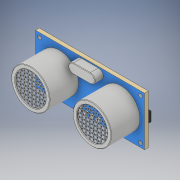
# Autodesk Inventor part: HC-SR04
Saved by Autodesk Inventor 2019 (Build 230136000, 136)
## iProperties
Created: 2020-12-06
Part Number: HC-SR04
Material: Типовые
Document SubType Name: Modeling
Designer: Professional
Density: 1 g/cm^3
Appearance: По умолчанию
Author: Professional
Autodesk Inventor part; units mm, degrees
note: some values were not read from the file. Chosen so that the rebuilt part matches the saved one: sketch regions of "Выдавливание1".
ref_plane "YZ Plane" through (0, 0, 0) normal (1, 0, 0) x (0, 1, 0)
ref_plane "XZ Plane" through (0, 0, 0) normal (0, 1, 0) x (-1, 0, 0)
ref_plane "XY Plane" through (0, 0, 0) normal (0, 0, 1) x (1, 0, 0)
sketch "Эскиз1" plane through (0, 0, 0) normal (0, 0, 1) x (1, 0, 0)
  line L0 (-22.7, -10.2) -> (22.7, -10.2)
  line L1 (22.7, -10.2) -> (22.7, 10.2)
  line L2 (22.7, 10.2) -> (-22.7, 10.2)
  line L3 (-22.7, 10.2) -> (-22.7, -10.2)
  line L4 (0, -10.2) -> (0, 10.2)
  circle A0 centre (-21, 8.5) radius 0.8
  circle A1 centre (-21, -8.5) radius 0.8
  circle A2 centre (21, 8.5) radius 0.8
  circle A3 centre (21, -8.5) radius 0.8
  line L5 (-22.7, 0) -> (22.7, 0)
  point P0 (0, 0)
  dimension "d0" = 45.4
  dimension "d1" = 20.4
  dimension "d2" = 42
  dimension "d3" = 17
  dimension "d4" = 1.6
  constraints: 12 end point, 4 centre point, 4 midpoint, 2 parallel, 2 symmetric about line, 2 vertical alignment, 1 horizontal, 1 horizontal alignment, 1 perpendicular, 1 vertical, 3 other
  measures "d0" distance of L1.end L2.end
  measures "d1" distance between parallel lines of L0 L2
  measures "d2" diameter of A0.centre L4
  measures "d3" distance of A1.centre A0.centre
  measures "d4" diameter of A0
extrude "Выдавливание1" add sketch "Эскиз1" along normal blind 1.6
sketch "Эскиз2" plane through (0, 0, 1.6) normal (0, 0, 1) x (1, 0, 0)
  circle A0 centre (-12.8, 0) radius 8
  circle A1 centre (12.8, 0) radius 8
  line L0 (22.7, 10.2) -> (-22.7, 10.2) projected
  line L1 (0, 10.2) -> (0, -10.2)
  line L2 (-22.7, -10.2) -> (22.7, -10.2) projected
  point P0 (0, 0)
  point P1 (0, 0)
  dimension "d7" = 16
  dimension "d8" = 25.6
  constraints: 3 midpoint, 2 centre point, 2 end point, 1 horizontal alignment, 1 vertical, 1 other
  measures "d7" diameter of A1
  measures "d8" distance of A0.centre A1.centre
extrude "Выдавливание2" add sketch "Эскиз2" along normal blind 12
sketch "Эскиз3" plane through (-12.8, 0, 13.6) normal (0, 0, 1) x (1, 0, 0)
  circle A0 centre (0, 0) radius 6.4
  circle A1 centre (25.6, 0) radius 6.4
  circle A2 centre (25.6, 0) radius 8 projected
  circle A3 centre (0, 0) radius 8 projected
  point P0 (12.8, 0)
  dimension "d11" = 1.6
  constraints: 2 centre point, 2 coincident, 1 equal radius
  measures "d11" radial gap between concentric circles of A2 A1
extrude "Выдавливание3" cut sketch "Эскиз3" against normal blind 0.4 contours A0 | A1
chamfer "Фаска1" distance 0.2 angle 45 4 edges at (-20.8, 0, 13.6) (4.8, 0, 13.6) (-19.2, 0, 13.6) (6.4, 0, 13.6)
sketch "Эскиз4" plane through (0, 0, 1.6) normal (0, 0, 1) x (1, 0, 0)
  line L0 (3.5, 7.7) -> (-3.5, 7.7) construction
  line L1 (3.5, 9.7) -> (-3.5, 9.7)
  line L2 (-3.5, 5.7) -> (3.5, 5.7)
  arc A0 (3.5, 5.7) -> (3.5, 9.7) centre (3.5, 7.7) ccw
  arc A1 (-3.5, 9.7) -> (-3.5, 5.7) centre (-3.5, 7.7) ccw
  line L3 (22.7, 10.2) -> (-22.7, 10.2) projected
  point P0 (0, 0)
  point P1 (0, 7.7)
  dimension "d17" = 7
  dimension "d18" = 2
  dimension "d19" = 2.5
  constraints: 8 end point, 4 point on circle, 4 tangent, 2 centre point, 1 horizontal, 1 midpoint, 1 parallel, 1 vertical alignment
  measures "d17" distance of L0.start L0.end
  measures "d18" radius of A1
  measures "d19" distance between parallel lines of L3 L0
extrude "Выдавливание4" add sketch "Эскиз4" along normal blind 3.5
sketch "Эскиз5" plane through (0, 0, 1.6) normal (0, 0, 1) x (1, 0, 0)
  circle A0 centre (3.81, -8.7) radius 0.8
  circle A1 centre (1.27, -8.7) radius 0.8
  circle A2 centre (-1.27, -8.7) radius 0.8
  circle A3 centre (-3.81, -8.7) radius 0.8
  line L0 (0, 0) -> (0, -10.2)
  line L1 (-22.7, -10.2) -> (22.7, -10.2) projected
  dimension "d22" = 2.54
  dimension "d23" = 7.62
  dimension "d24" = 1.6
  dimension "d25" = 1.5
  constraints: 4 centre point, 2 end point, 1 equal radius, 1 horizontal alignment, 1 midpoint, 2 other
  measures "d22" distance of A2.centre A1.centre
  measures "d23" distance of A3.centre A0.centre
  measures "d24" diameter of A3
  measures "d25" distance from line of L1 A1.centre
extrude "Выдавливание5" add sketch "Эскиз5" along normal blind 1
fillet "Сопряжение1" radius 0.4 4 edges at (-4.61, -8.7, 2.6) (-2.07, -8.7, 2.6) (0.47, -8.7, 2.6) (3.01, -8.7, 2.6)
sketch "Эскиз7" plane through (0, 0, 0) normal (0, 0, -1) x (-1, 0, 0)
  line L0 (-22.2, 2) -> (-13.2, 2)
  line L1 (-13.2, 2) -> (-13.2, -2)
  line L2 (-13.2, -2) -> (-22.2, -2)
  line L3 (-22.2, -2) -> (-22.2, 2)
  line L4 (20.7, 4.5) -> (16.7, 4.5)
  line L5 (16.7, 4.5) -> (16.7, -4.5)
  line L6 (16.7, -4.5) -> (20.7, -4.5)
  line L7 (20.7, -4.5) -> (20.7, 4.5)
  line L8 (-4.5, 2) -> (4.5, 2)
  line L9 (4.5, 2) -> (4.5, -2)
  line L10 (4.5, -2) -> (-4.5, -2)
  line L11 (-4.5, -2) -> (-4.5, 2)
  line L12 (22.7, 10.2) -> (22.7, -10.2) projected
  line L13 (-22.7, -10.2) -> (-22.7, 10.2) projected
  point P0 (0, 0)
  point P1 (0, -2)
  point P2 (-4.5, 0)
  point P3 (16.7, 0)
  dimension "d31" = 9
  dimension "d32" = 4
  dimension "d33" = 2
  dimension "d34" = 0.5
  constraints: 24 end point, 6 parallel, 3 equal length, 3 horizontal, 3 midpoint, 3 perpendicular, 2 horizontal alignment, 2 point on line, 1 vertical alignment
  measures "d31" distance of L8.start L8.end
  measures "d32" distance between parallel lines of L10 L8
  measures "d33" distance between parallel lines of L12 L7
  measures "d34" distance between parallel lines of L13 L3
extrude "Выдавливание7" add sketch "Эскиз7" along normal blind 1.6
sketch "Эскиз8" plane through (0, 0, 0) normal (0, 0, -1) x (-1, 0, 0)
  circle A0 centre (12.8, 0) radius 8 projected
  circle A1 centre (12.8, 0) radius 8 projected
  line L0 (22.7, -10.2) -> (-22.7, -10.2) projected
  line L1 (0, -10.2) -> (0, 10.2)
  line L2 (-22.7, 10.2) -> (22.7, 10.2) projected
  circle A2 centre (12.8, 5) radius 1
  circle A3 centre (12.8, -5) radius 1
  circle A4 centre (12.8, 0) radius 5 construction
  circle A5 centre (-12.8, 5) radius 1
  circle A6 centre (-12.8, -5) radius 1
  point P0 (0, 0)
  dimension "d37" = 10
  dimension "d38" = 2
  constraints: 5 centre point, 2 end point, 2 midpoint, 2 point on circle, 2 symmetric about line, 2 vertical alignment, 1 coincident, 1 equal radius, 2 other
  measures "d37" distance of A2.centre A3.centre
  measures "d38" diameter of A2
extrude "Выдавливание8" add sketch "Эскиз8" along normal blind 1.3 contours A2 | A3 | A5 | A6
chamfer "Фаска2" distance 0.2 angle 45 4 edges at (0, 9.7, 5.1) (-5.5, 7.7, 5.1) (0, 5.7, 5.1) (5.5, 7.7, 5.1)
sketch "Эскиз9" plane through (0, 0, 0) normal (0, 0, -1) x (-1, 0, 0)
  circle A0 centre (3.81, -8.7) radius 0.8 projected
  circle A1 centre (3.81, -8.7) radius 0.8 projected
  circle A2 centre (1.27, -8.7) radius 0.8 projected
  circle A3 centre (1.27, -8.7) radius 0.8 projected
  circle A4 centre (-1.27, -8.7) radius 0.8 projected
  circle A5 centre (-1.27, -8.7) radius 0.8 projected
  circle A6 centre (-3.81, -8.7) radius 0.8 projected
  line L0 (-5.5, -7.3) -> (5.5, -7.3)
  line L1 (5.5, -7.3) -> (5.5, -10.1)
  line L2 (5.5, -10.1) -> (-5.5, -10.1)
  line L3 (-5.5, -10.1) -> (-5.5, -7.3)
  line L4 (-4.5, -2) -> (4.5, -2) projected
  line L5 (22.7, -10.2) -> (-22.7, -10.2) projected
  point P0 (0, 0)
  point P1 (0, -7.3)
  point P2 (0, -2)
  dimension "d44" = 0.1
  dimension "d45" = 11
  dimension "d46" = 2.8
  constraints: 8 end point, 2 midpoint, 2 parallel, 1 horizontal, 1 perpendicular, 1 vertical alignment
  measures "d44" distance between parallel lines of L2 L5
  measures "d45" distance between parallel lines of L1 L3
  measures "d46" distance between parallel lines of L2 L0
extrude "Выдавливание9" add sketch "Эскиз9" along normal blind 2.4 contours A0 | A2 | A4 | A6 | L0 L1 L2 L3
chamfer "Фаска3" distance 0.6 angle 45 4 edges at (-5.5, -10.1, -1.2) (-5.5, -7.3, -1.2) (5.5, -7.3, -1.2) (5.5, -10.1, -1.2)
sketch "Эскиз10" plane through (0, 0, -2.4) normal (0, 0, -1) x (-1, 0, 0)
  circle A0 centre (-3.81, -8.7) radius 0.8 construction
  circle A1 centre (-1.27, -8.7) radius 0.8 construction
  circle A2 centre (1.27, -8.7) radius 0.8 construction
  circle A3 centre (3.81, -8.7) radius 0.8 construction
  circle A4 centre (-3.81, -8.7) radius 0.8 projected
  line L0 (-4.3757, -9.2657) -> (-3.2443, -9.2657)
  line L1 (-3.2443, -9.2657) -> (-3.2443, -8.1343)
  line L2 (-3.2443, -8.1343) -> (-4.3757, -8.1343)
  line L3 (-4.3757, -8.1343) -> (-4.3757, -9.2657)
  line L4 (-4.3757, -9.2657) -> (-3.2443, -8.1343) construction
  line L5 (-3.2443, -9.2657) -> (-4.3757, -8.1343) construction
  line L6 (-1.8357, -9.2657) -> (-0.7043, -9.2657)
  line L7 (-0.7043, -9.2657) -> (-0.7043, -8.1343)
  line L8 (-0.7043, -8.1343) -> (-1.8357, -8.1343)
  line L9 (-1.8357, -8.1343) -> (-1.8357, -9.2657)
  line L10 (-1.8357, -9.2657) -> (-0.7043, -8.1343) construction
  line L11 (-0.7043, -9.2657) -> (-1.8357, -8.1343) construction
  line L12 (0.7043, -9.2657) -> (1.8357, -9.2657)
  line L13 (1.8357, -9.2657) -> (1.8357, -8.1343)
  line L14 (1.8357, -8.1343) -> (0.7043, -8.1343)
  line L15 (0.7043, -8.1343) -> (0.7043, -9.2657)
  line L16 (0.7043, -9.2657) -> (1.8357, -8.1343) construction
  line L17 (1.8357, -9.2657) -> (0.7043, -8.1343) construction
  line L18 (3.2443, -9.2657) -> (4.3757, -9.2657)
  line L19 (4.3757, -9.2657) -> (4.3757, -8.1343)
  line L20 (4.3757, -8.1343) -> (3.2443, -8.1343)
  line L21 (3.2443, -8.1343) -> (3.2443, -9.2657)
  line L22 (3.2443, -9.2657) -> (4.3757, -8.1343) construction
  line L23 (4.3757, -9.2657) -> (3.2443, -8.1343) construction
  point P0 (0, 0)
  constraints: 48 end point, 8 midpoint, 8 parallel, 5 perpendicular, 4 horizontal, 3 point on line, 1 point on circle, 6 other
extrude "Выдавливание10" add sketch "Эскиз10" along normal blind 8 contours L1 L0 L3 L2 | L9 L8 L7 L6 | L15 L14 L13 L12 | L21 L20 L19 L18
chamfer "Фаска4" distance 0.4 angle 45 16 edges at (4.3757, -8.7, -10.4) (3.2443, -8.7, -10.4) (1.8357, -8.7, -10.4) (0.7043, -8.7, -10.4) (1.27, -8.1343, -10.4) (1.27, -9.2657, -10.4) (3.81, -8.1343, -10.4) (3.81, -9.2657, -10.4) (-1.27, -9.2657, -10.4) (-0.7043, -8.7, -10.4) (-1.27, -8.1343, -10.4) (-1.8357, -8.7, -10.4) (-3.2443, -8.7, -10.4) (-3.81, -9.2657, -10.4) (-4.3757, -8.7, -10.4) (-3.81, -8.1343, -10.4)
chamfer "Фаска5" distance 0.4 angle 45 4 edges at (13.8, -5, -1.3) (13.8, 5, -1.3) (-11.8, -5, -1.3) (-11.8, 5, -1.3)
